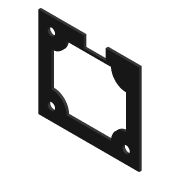
# Autodesk Inventor part: resin_bottom
Saved by Autodesk Inventor 2015 SP1 (Build 190203100, 203)
## iProperties
Created: 2015-12-07
Part Number: resin_bottom
Material: Generic
Document SubType Name: Modeling
Designer: User
Density: 1 g/cm^3
Appearance: Default
Mass: 0.737523 g
Surface Area: 17.6395 cm^2
Volume: 0.737523 cm^3
Author: User
Autodesk Inventor part; units mm, degrees
ref_plane "YZ Plane" through (0, 0, 0) normal (1, 0, 0) x (0, 1, 0)
ref_plane "XZ Plane" through (0, 0, 0) normal (0, 1, 0) x (-1, 0, 0)
ref_plane "XY Plane" through (0, 0, 0) normal (0, 0, 1) x (1, 0, 0)
sketch "Эскиз1" plane through (0, 0, 0) normal (0, 1, 0) x (-1, 0, 0)
  line L0 (18, -16) -> (-18, -16)
  line L1 (-18, -16) -> (-18, 16)
  line L2 (-18, 16) -> (18, 16)
  line L3 (18, 16) -> (18, -16)
  line L4 (0, -25.2) -> (0, 25.2)
  line L5 (28, 0) -> (-28, 0)
  line L6 (14.82, -12.82) -> (-14.82, -12.82)
  line L7 (-14.82, -12.82) -> (-14.82, 12.82)
  line L8 (-14.82, 12.82) -> (14.82, 12.82)
  line L9 (14.82, 12.82) -> (14.82, -12.82)
  circle A0 centre (14.82, -12.82) radius 1.5
  circle A1 centre (14.82, 12.82) radius 1.5
  circle A2 centre (-14.82, 12.82) radius 1.5
  circle A3 centre (-14.82, -12.82) radius 1.5
  arc A4 (14.82, -6.82) -> (8.82, -12.82) centre (14.82, -12.82) ccw
  arc A5 (-8.82, -12.82) -> (-14.82, -6.82) centre (-14.82, -12.82) ccw
  arc A6 (8.82, 12.82) -> (14.82, 6.82) centre (14.82, 12.82) ccw
  arc A7 (-14.82, 6.82) -> (-8.824, 12.6) centre (-14.82, 12.82) ccw
  line L10 (20, -18) -> (-20, -18)
  line L11 (-20, -18) -> (-20, 18)
  line L12 (-20, 18) -> (20, 18)
  line L13 (20, 18) -> (20, -18)
  line L14 (-8.82, -12.82) -> (-8.82, -16)
  line L15 (8.82, -12.82) -> (8.82, -16)
  line L16 (14.82, -6.82) -> (18, -6.82)
  line L17 (14.82, 6.82) -> (18, 6.82)
  line L18 (-14.82, -6.82) -> (-20, -6.82)
  line L19 (-14.82, 6.82) -> (-20, 6.82)
  line L20 (-8.82, 12.82) -> (-8.82, 18)
  line L21 (-18, -6.82) -> (-18, 6.82)
  line L22 (8.82, 16) -> (-8.82, 16)
  line L23 (2, 13.6) -> (-6.7, 13.6)
  line L24 (-6.7, 13.6) -> (-6.7, 18)
  line L25 (3.5, 16) -> (3.5, 12.6)
  line L26 (3.5, 12.6) -> (-8.2, 12.6)
  line L27 (-8.2, 12.6) -> (-8.2, 16)
  line L28 (2, 13.6) -> (2, 18)
  line L29 (3.5, 16) -> (2, 16)
  line L30 (2, 16) -> (2, 18)
  line L31 (14.82, 6.82) -> (18, 6.82)
  line L32 (8.82, 12.82) -> (8.82, 16)
  line L33 (-8.2, 12.6) -> (-8.824, 12.6)
  line L34 (3.5, 12.6) -> (8.824, 12.6)
  line L35 (8.824, 12.6) -> (8.824, 12.82)
  line L36 (8.824, 12.82) -> (3.5, 12.82)
  line L37 (3.5, 12.82) -> (3.5, 12.6)
  point P0 (0, 0)
  point P1 (0, 0)
  point P2 (-13.034, 10.913)
  dimension "d0" = 36
  dimension "d1" = 32
  dimension "d2" = 3.18
  dimension "d3" = 3.18
  dimension "d4" = 3.18
  dimension "d5" = 3.18
  dimension "d6" = 3
  dimension "d7" = 3
  dimension "d8" = 3
  dimension "d9" = 3
  dimension "d10" = 12
  dimension "d11" = 12
  dimension "d12" = 12
  dimension "d13" = 12
  dimension "d14" = 4.966
  dimension "d15" = 5.087
  dimension "d16" = 2
  dimension "d17" = 2
  dimension "d18" = 2
  dimension "d19" = 2
  dimension "d20" = 11.3
  dimension "d21" = 2.4
  dimension "d22" = 1
  dimension "d23" = 1.5
  dimension "d24" = 1.5
  dimension "d25" = 16
  constraints: 76 end point, 33 point on line, 17 perpendicular, 9 point on circle, 8 centre point, 8 coincident, 7 parallel, 5 horizontal, 3 tangent, 1 collinear, 1 vertical, 2 other
  measures "d0" distance of L0.start L0.end
  measures "d1" distance of L0.end L1.end
  measures "d2" distance between parallel lines of L3 L9
  measures "d3" distance between parallel lines of L2 L8
  measures "d4" distance between parallel lines of L1 L7
  measures "d5" distance between parallel lines of L0 L6
  measures "d6" diameter of A0
  measures "d7" diameter of A1
  measures "d8" diameter of A2
  measures "d9" diameter of A3
  measures "d10" diameter of A4
  measures "d11" diameter of A5
  measures "d12" diameter of A6
  measures "d13" diameter of A7
  measures "d14" distance from line of L1 point (-13.034, 10.913)
  measures "d15" distance from line of L2 point (-13.034, 10.913)
  measures "d16" distance between parallel lines of L10 L0
  measures "d17" distance between parallel lines of L13 L3
  measures "d18" distance between parallel lines of L2 L12
  measures "d19" distance between parallel lines of L11 L1
  measures "d20" distance between parallel lines of L1 L24
  measures "d21" distance between parallel lines of L22 L23
  measures "d22" distance between parallel lines of L26 L23
  measures "d23" distance between parallel lines of L24 L27
  measures "d24" distance between parallel lines of L25 L28
  measures "d25" distance between parallel lines of L3 L28
extrude "Выдавливание1" add sketch "Эскиз1" along normal blind 1 contours L3 L5 L13 L10 L4 L0 | L0 L15 L6 A0 L9 L16 L3 | L0 L4 L6 L15 | L16 L9 L5 L3 | L4 L10 L11 L18 L1 L0 | L0 L14 L6 L4 | A4 L9 A0 L6 | L5 L9 L17 L3 | L3 L2 L28 L12 L13 L5 | L0 L1 L18 L7 A3 L6 L14 | A0 L9 L6 | L6 L9 A0 | L17 L9 A1 L8 L32 L2 L3 | L6 A3 L7 A5 | A6 L35 L8 A1 L9 | L18 L11 L5 L1 | L1 L5 L7 L18 | A3 L7 L6 | L6 L7 A3 | L26 L27 L8 L4 | L4 L8 L25 L26 | L5 L1 L19 L7 | L32 L8 L25 L2 | A1 L8 L9 | L9 L8 A1 | L34 L25 L8 A6 | A6 L8 L35 | L5 L11 L19 L1 | L8 L27 L2 L24 L23 L4 | L4 L23 L28 L2 L25 L8 | L33 A7 L7 A2 L8 L27 | L19 L1 L2 L20 L8 A2 L7 | L19 L11 L12 L20 L2 L1 | L8 L20 L2 L27 | A2 L8 L7 | L7 L8 A2 | L24 L2 L20 L12
extrude "Выдавливание2" cut sketch "Эскиз1" along normal up to next contours A0 L9 L6 | L6 L9 A0 | A3 L7 L6 | L6 L7 A3 | A1 L8 L9 | L9 L8 A1
equation "\"d6\" = d9"
equation "\"d7\" = d9"
equation "\"d8\" = d9"
